snowboard (Autodesk Fusion 360 design; units mm, degrees)
Autodesk Fusion 360 part; units mm, degrees
sketch "Sketch1" plane through (0, 0, 0) normal (0, 0, 1) x (1, 0, 0)
  arc A0 (17.6, -8.5) -> (17.6, 8.5) centre (17.6, 0) ccw
  arc A1 (0, 8.5) -> (0, -8.5) centre (0, 0) ccw
  line L0 (0, 0) -> (17.6, 0) construction
  circle A2 centre (8.8, 0) radius 7.5
  circle A3 centre (17.6, 0) radius 1.25
  circle A4 centre (0, 0) radius 1.25
  circle A5 centre (8.8, 0) radius 6.5
  line L1 (4.8, -8.5) -> (4.8, -13)
  line L2 (5.8, -14) -> (11.8, -14)
  line L3 (12.8, -13) -> (12.8, -8.5)
  arc A6 (4.8, -13) -> (5.8, -14) centre (5.8, -13) ccw
  arc A7 (11.8, -14) -> (12.8, -13) centre (11.8, -13) ccw
  line L4 (0, -8.5) -> (4.8, -8.5)
  line L5 (12.8, -8.5) -> (17.6, -8.5)
  line L6 (12.8, 13) -> (12.8, 8.5)
  arc A8 (12.8, 13) -> (11.8, 14) centre (11.8, 13) ccw
  line L7 (5.8, 14) -> (11.8, 14)
  arc A9 (5.8, 14) -> (4.8, 13) centre (5.8, 13) ccw
  line L8 (4.8, 8.5) -> (4.8, 13)
  line L9 (17.6, 8.5) -> (12.8, 8.5)
  line L10 (4.8, 8.5) -> (0, 8.5)
  line L11 (12.8, 8.5) -> (4.8, 8.5)
  line L12 (4.8, -8.5) -> (12.8, -8.5)
  point P0 (8.8, -8.5)
  point P1 (12.8, -14)
  dimension "d1" = 17
  dimension "d2" = 15
  dimension "d3" = 2.5
  dimension "d4" = 2.5
  dimension "d5" = -1
  dimension "d26" = 4
  dimension "d27" = 8
  dimension "d28" = 5.5
  dimension "d29" = 1
  constraint tangent A0 L4
  constraint tangent A0 L9
  constraint parallel L4 L9
  constraint tangent A1 L9
  constraint tangent A1 L4
  constraint horizontal L0
  constraint coincident A1.centre L0.start
  constraint midpoint L0 A2.centre
  constraint concentric A0 A3
  constraint concentric A1 A4
  constraint vertical L1
  constraint horizontal L2
  constraint vertical L3
  constraint tangent L1 A6
  constraint tangent L2 A6
  constraint coincident P1 L2
  constraint coincident P1 L3
  constraint tangent L2 A7
  constraint tangent L3 A7
  constraint equal A6 A7
  constraint collinear L4 L5
  constraint coincident P0 L4
  constraint symmetric L0 L3.end L6.end
  constraint symmetric L0 L1.start L8.start
  constraint symmetric L0 L1.end A9.end
  constraint symmetric L0 L2.start L7.start
  constraint symmetric L0 A6 A9
  constraint symmetric L0 L2.end A8.end
  constraint symmetric L0 L3.start L6.start
  constraint symmetric L0 A7 A8
  constraint tangent A1 L10
  measures "d1" diameter of A0
  measures "d2" diameter of A2
  measures "d3" diameter of A3
  measures "d4" diameter of A4
  measures "d26" distance of P0 L3.end
  measures "d27" distance of L3.end L1.start
  measures "d28" distance of L3.end P1
  measures "d29" radius of A6
extrude "Extrude1" add sketch "Sketch1" along normal blind 45 contours A2
extrude "Extrude2" add sketch "Sketch1" along normal blind 2 contours A0 A1 L4 L5 L9 L10 L11 L12
extrude "Extrude3" add sketch "Sketch1" along normal blind 0.1 contours A3 | A4
fillet "Fillet1" radius 0.2 4 edges at (-8.5, 0, 0) (8.8, -8.5, 0) (26.1, 0, 0) (8.8, 8.5, 0)
fillet "Fillet2" radius 0.5 1 edges at (1.8075, -2.7121, 45)
fillet "Fillet3" radius 0.2 1 edges at (-1.1654, 0.452, 2)
fillet "Fillet4" radius 0.2 1 edges at (16.4346, 0.452, 2)
fillet "Fillet5" radius 0.2 1 edges at (1.8075, -2.7121, 2)
fillet "Fillet6" [suppressed]
extrude "Extrude4" add sketch "Sketch1" along normal blind 1.5 contours A5
sketch "Sketch2" plane through (0, 0, 2) normal (0, 0, 1) x (-1, 0, 0)
  arc A0 (-1.1507, 0.8823) -> (-16.4493, 0.8823) centre (-8.8, 0) ccw
  arc A1 (-1.1507, -0.8823) -> (-1.1507, 0.8823) centre (0, 0) ccw
  arc A2 (-16.4493, -0.8823) -> (-1.1507, -0.8823) centre (-8.8, 0) ccw
  arc A3 (-16.4493, 0.8823) -> (-16.4493, -0.8823) centre (-17.6, 0) ccw
  line L0 (0, 8.5) -> (-17.6, 8.5)
  arc A4 (-17.6, 8.5) -> (-17.6, -8.5) centre (-17.6, 0) ccw
  line L1 (-17.6, -8.5) -> (0, -8.5)
  arc A5 (0, -8.5) -> (0, 8.5) centre (0, 0) ccw
extrude "Extrude5" add sketch "Sketch1" along normal blind 3 contours L1 L2 L3 A6 A7 L12 | L6 A8 L7 A9 L8 L11
extrude "Extrude6" cut sketch "Sketch1" along normal blind 1 contours L1 L2 L3 A6 A7 L12 | L6 A8 L7 A9 L8 L11
fillet "Fillet10" radius 0.5 1 edges at (8.8, -8.5, 2)
fillet "Fillet11" radius 0.5 1 edges at (8.8, 8.5, 2)
fillet "Fillet12" radius 0.1 1 faces at (9.8, 10.3333, 3)
fillet "Fillet13" radius 0.5 1 edges at (8.8, -8.5, 1)
fillet "Fillet14" radius 0.1 1 faces at (7.8, -10.3333, 3)
fillet "Fillet15" radius 0.5 1 edges at (8.8, 8.5, 1)
fillet "Fillet16" radius 0.1 7 edges at (12.8, 8.6464, 0.8536) (12.8, 11, 1) (12.5071, 13.7071, 1) (8.8, 14, 1) (5.0929, 13.7071, 1) (4.8, 11, 1) (4.8, 8.6464, 0.8536)
fillet "Fillet17" radius 0.1 7 edges at (4.8, -8.6464, 0.8536) (4.8, -11, 1) (5.0929, -13.7071, 1) (8.8, -14, 1) (12.5071, -13.7071, 1) (12.8, -11, 1) (12.8, -8.6464, 0.8536)
